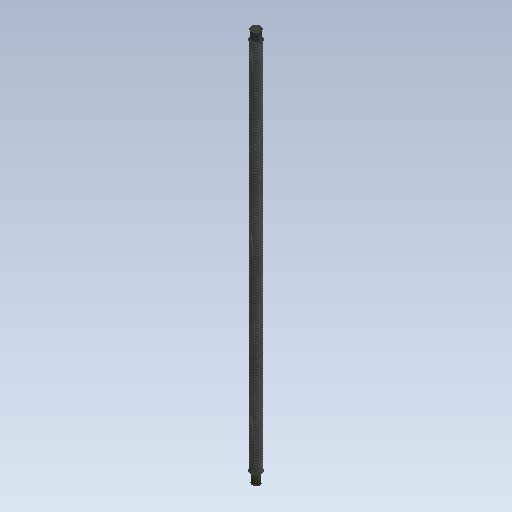
# Autodesk Inventor part: Tornillo de mesa
Saved by Autodesk Inventor 2020 (Build 240168000, 168)
## iProperties
Created: 2020-05-16
Part Number: Tornillo de mesa
Material: Steel
Document SubType Name: Modeling
Designer: Pipi
Density: 7.85 g/cm^3
Appearance: Plate
Mass: 47.8779 g
Surface Area: 162.86 cm^2
Volume: 47.8779 cm^3
Author: Pipi
Autodesk Inventor part; units mm, degrees
ref_plane "YZ Plane" through (0, 0, 0) normal (1, 0, 0) x (0, 1, 0)
ref_plane "XZ Plane" through (0, 0, 0) normal (0, 1, 0) x (-1, 0, 0)
ref_plane "XY Plane" through (0, 0, 0) normal (0, 0, 1) x (1, 0, 0)
sketch "Boceto1" plane through (0, 0, 0) normal (0, 1, 0) x (-1, 0, 0)
  circle A0 centre (4.7317, 15.3673) radius 6
  point P0 (0, 0)
  dimension "d0" = 12
  constraints: 1 centre point
  measures "d0" diameter of A0
extrude "Extrusión1" add sketch "Boceto1" along normal blind 434
thread "Rosca1" size "M12x1.5" class "6g" standard "ANSI Metric M Profile" length 430
sketch "Sketch2" plane through (-4.7317, 0, 15.3673) normal (0, -1, 0) x (1, 0, 0)
  circle A0 centre (0, 0) radius 4
  circle A1 centre (0, 0) radius 6
  dimension "d5" = 8
  constraints: 2 centre point, 1 coincident
  measures "d5" diameter of A0
extrude "Extrusion2" cut sketch "Sketch2" against normal blind 12
sketch "Sketch3" plane through (-4.7317, 434, 15.3673) normal (0, 1, 0) x (1, 0, 0)
  circle A0 centre (0, 0) radius 5
  circle A1 centre (0, 0) radius 6
  dimension "d8" = 10
  constraints: 2 centre point, 1 coincident
  measures "d8" diameter of A0
extrude "Extrusion3" cut sketch "Sketch3" against normal blind 10
